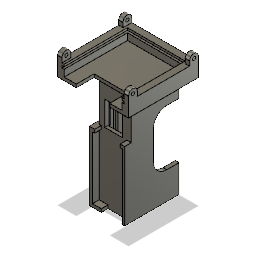
TinyTrack v7 (Autodesk Fusion 360 design; units mm, degrees)
Autodesk Fusion 360 part; units mm, degrees
sketch "Sketch1" plane through (0, 0, 0) normal (0, 1, 0) x (1, 0, 0)
  line L0 (0, 0) -> (26, 0)
  line L1 (26, 0) -> (26, 28.5)
  line L2 (26, 28.5) -> (0, 28.5)
  line L3 (0, 28.5) -> (0, 0)
  line L4 (29, -3) -> (29, 31.5)
  line L5 (29, 31.5) -> (-3, 31.5)
  line L6 (-3, 31.5) -> (-3, -3)
  line L7 (-3, -3) -> (29, -3)
  line L8 (27, -1) -> (27, 29.5)
  line L9 (27, 29.5) -> (-1, 29.5)
  line L10 (-1, 29.5) -> (-1, -1)
  line L11 (-1, -1) -> (27, -1)
  line L12 (-1, -1) -> (-1, -3)
  line L13 (27, -1) -> (27, -3)
  line L14 (0, 0) -> (0, -1)
  line L15 (26, 0) -> (26, -1)
  line L16 (0, -1) -> (0, -3)
  line L17 (26, -1) -> (26, -3)
  line L18 (5.5, -3) -> (20.5, -3)
  line L19 (20.5, -3) -> (20.5, 8)
  line L20 (20.5, 8) -> (5.5, 8)
  line L21 (5.5, 8) -> (5.5, -3)
  line L22 (7.5, 31.5) -> (18.5, 31.5)
  line L23 (18.5, 31.5) -> (18.5, 11.5)
  line L24 (18.5, 11.5) -> (7.5, 11.5)
  line L25 (7.5, 11.5) -> (7.5, 31.5)
  line L26 (20.25, 31.5) -> (20.25, 10)
  line L27 (20.25, 10) -> (5.75, 10)
  line L28 (5.75, 10) -> (5.75, 31.5)
  line L29 (26, 28.5) -> (26, 29.5)
  line L30 (0, 28.5) -> (0, 29.5)
  line L31 (7.5, 15.5) -> (8.75, 15.5)
  line L32 (8.75, 15.5) -> (8.75, 17.5)
  line L33 (8.75, 17.5) -> (7.5, 17.5)
  line L34 (7.5, 17.5) -> (7.5, 15.5)
  line L35 (18.5, 15.5) -> (17.25, 15.5)
  line L36 (17.25, 15.5) -> (17.25, 17.5)
  line L37 (17.25, 17.5) -> (18.5, 17.5)
  line L38 (18.5, 17.5) -> (18.5, 15.5)
  line L39 (7.5, 11.5) -> (8.75, 11.5)
  line L40 (8.75, 11.5) -> (8.75, 13.5)
  line L41 (8.75, 13.5) -> (7.5, 13.5)
  line L42 (7.5, 13.5) -> (7.5, 11.5)
  line L43 (18.5, 11.5) -> (17.25, 11.5)
  line L44 (17.25, 11.5) -> (17.25, 13.5)
  line L45 (17.25, 13.5) -> (18.5, 13.5)
  line L46 (18.5, 13.5) -> (18.5, 11.5)
  line L47 (26, 0) -> (29, 0)
  line L48 (0, 0) -> (-3, 0)
  dimension "d1" = 26
  dimension "d2" = 28.5
  dimension "d3" = 3
  dimension "d4" = 1
  dimension "d15" = 15
  dimension "d16" = 11
  dimension "d17" = 5.5
  dimension "d18" = 11
  dimension "d19" = 20
  dimension "d21" = 1.25
  dimension "d22" = 2
  dimension "d23" = 2
  dimension "d24" = 1.25
  dimension "d25" = 4
  dimension "d26" = 4
  dimension "d42" = 1.25
  dimension "d43" = 2
  dimension "d44" = 2
  dimension "d45" = 1.25
  dimension "d56" = 1.75
  dimension "d57" = 1.75
  dimension "d58" = 8.75
  measures "d17" distance of L3 L21
  measures "d25" distance of L24 L31
  measures "d26" distance of L24 L35
  measures "d56" distance of L23 L26
  measures "d57" distance of L25 L28
  measures "d58" distance of L4 L26
extrude "Extrude1" add sketch "Sketch1" along normal blind 1.5 contours L0 L1 L2 L3 L19 L20 L21 L26 L27 L28 | L2 L23 L24 L25 L26 L27 L28 L34 L38 L39 L42 L43 L46 | L2 L23 L24 L25 L31 L32 L33 L35 L36 L37 L40 L41 L44 L45 | L25 L31 L32 L33 L34 | L23 L35 L36 L37 L38 | L24 L25 L39 L40 L41 L42 | L23 L24 L43 L44 L45 L46
extrude "Extrude2" add sketch "Sketch1" along normal blind 4.5 contours L3 L9 L10 L30 L48 | L2 L9 L28 L30 | L2 L9 L25 L28 | L1 L8 L9 L29 L47 | L2 L9 L23 L25 | L2 L9 L26 L29 | L2 L9 L23 L26
extrude "Extrude3" add sketch "Sketch1" along normal blind 6.5 contours L5 L6 L9 L10 L28 L48 | L5 L9 L25 L28 | L4 L5 L8 L9 L26 L47 | L5 L9 L22 L23 L25 | L5 L9 L23 L26
extrude "Extrude4" add sketch "Sketch1" along normal blind 1 from surface at 5.5 contours L3 L9 L10 L30 L48 | L2 L9 L28 L30 | L2 L9 L25 L28 | L1 L8 L9 L29 L47 | L2 L9 L23 L25 | L2 L9 L26 L29 | L2 L9 L23 L26
extrude "Extrude5" add sketch "Sketch1" against normal blind 50 contours L2 L9 L25 L28 | L2 L23 L24 L25 L26 L27 L28 L34 L38 L39 L42 L43 L46 | L5 L9 L25 L28 | L2 L9 L23 L26 | L25 L31 L32 L33 L34 | L5 L9 L23 L26 | L23 L35 L36 L37 L38 | L24 L25 L39 L40 L41 L42 | L23 L24 L43 L44 L45 L46
sketch "Sketch2" plane through (20.25, 0, 0) normal (1, 0, 0) x (0, 0, -1)
  line L0 (31.5, 0) -> (10, 0)
  line L1 (10, 0) -> (10, -50)
  line L2 (10, -50) -> (31.5, -50)
  line L3 (31.5, -50) -> (31.5, 0)
  line L4 (31.5, -12.5) -> (26, -12.5)
  line L5 (20, -18.5) -> (20, -31.5)
  line L6 (26, -37.5) -> (31.5, -37.5)
  line L7 (31.5, -37.5) -> (31.5, -12.5)
  arc A0 (26, -12.5) -> (20, -18.5) centre (26, -18.5) ccw
  arc A1 (20, -31.5) -> (26, -37.5) centre (26, -31.5) ccw
  dimension "d29" = 25
  dimension "d30" = 11.5
  dimension "d31" = 12.5
  dimension "d32" = 6
  dimension "d33" = 6
  measures "d29" distance of L4 L6
  measures "d30" distance of L5 L7
  measures "d31" distance of L0 L4
  measures "d32" radius of A0
  measures "d33" radius of A1
extrude "Extrude6" cut sketch "Sketch2" against normal blind 15 contours L3 L4 L5 L6 L7 A0 A1
sketch "Sketch3" plane through (0, 0, -10) normal (0, 0, 1) x (1, 0, 0)
  line L0 (20.25, 0) -> (5.75, 0)
  line L1 (5.75, 0) -> (5.75, -50)
  line L2 (5.75, -50) -> (20.25, -50)
  line L3 (20.25, -50) -> (20.25, 0)
  line L4 (8.25, -8) -> (16.25, -8)
  line L5 (16.25, -8) -> (16.25, -19)
  line L6 (16.25, -19) -> (8.25, -19)
  line L7 (8.25, -19) -> (8.25, -8)
  line L8 (21, -50) -> (21, -22)
  line L9 (5.75, -22) -> (5.75, -50)
  line L10 (5.75, -48.5) -> (21, -48.5)
  line L11 (21, -48.5) -> (21, -20.5)
  line L12 (21, -20.5) -> (5.75, -20.5)
  line L13 (5.75, -20.5) -> (5.75, -48.5)
  line L14 (5.75, -19) -> (19.25, -19)
  line L15 (19.25, -19) -> (20.75, -19)
  line L16 (20.75, -19) -> (20.75, -50)
  line L17 (20.75, -50) -> (19.25, -50)
  line L18 (19.25, -50) -> (19.25, -19)
  line L19 (5.75, -19) -> (4.25, -19)
  line L20 (4.25, -19) -> (4.25, -50)
  line L21 (4.25, -50) -> (5.75, -50)
  line L22 (5.75, -50) -> (5.75, -19)
  line L23 (9.75, -48.5) -> (9.75, -50)
  line L24 (18.25, -19) -> (18.25, -20.5)
  line L25 (6.75, -19) -> (6.75, -20.5)
  dimension "d36" = 8
  dimension "d37" = 11
  dimension "d38" = 8
  dimension "d39" = 2.5
  dimension "d61" = 28
  dimension "d62" = 1.5
  dimension "d63" = 13.5
  dimension "d64" = 1.5
  dimension "d65" = 1.5
  dimension "d66" = 1.5
  dimension "d67" = 1
  dimension "d69" = 1
  measures "d38" distance of L0 L4
  measures "d39" distance of L1 L7
  measures "d62" distance of L2 L10
  measures "d64" distance of L12 L14
  measures "d67" distance of L18 L24
  measures "d69" distance of L22 L25
extrude "Extrude7" cut sketch "Sketch3" against normal blind 2 contours L4 L5 L6 L7 L14
extrude "Extrude8" add sketch "Sketch3" against normal blind 2 contours L1 L12 L14 L22 L25 | L1 L9 L13 L19 L20 L21 L22 | L12 L14 L18 L24 | L1 L2 L9 L10 L22 L23
extrude "Extrude9" add sketch "Sketch3" along normal blind 3 contours L3 L12 L15 L18 | L1 L12 L14 L22 L25 | L1 L9 L13 L19 L20 L21 L22 | L3 L10 L12 L18 | L12 L14 L18 L24 | L2 L3 L10 L17 L18 | L1 L2 L9 L10 L22 L23
sketch "Sketch4" plane through (-3, 0, 0) normal (-1, 0, 0) x (0, 0, 1)
  line L0 (-31.5, 0) -> (0, 0)
  line L1 (0, 0) -> (0, 6.5)
  line L2 (0, 6.5) -> (-31.5, 6.5)
  line L3 (-31.5, 6.5) -> (-31.5, 0)
  line L4 (-31.5, 6.5) -> (-27.5, 6.5)
  line L5 (-27.5, 6.5) -> (-27.5, 8.5)
  line L6 (-31.5, 8.5) -> (-31.5, 8.5)
  line L7 (-31.5, 7.5) -> (-31.5, 6.5)
  line L8 (0, 6.5) -> (-4, 6.5)
  line L9 (-4, 6.5) -> (-4, 8.5)
  line L10 (-4, 8.4862) -> (-4, 8.4862)
  line L11 (0, 8.5) -> (0, 6.5)
  circle A0 centre (-29.5, 8.5) radius 0.75
  arc A1 (-27.5, 8.5) -> (-31.5, 8.5) centre (-29.5, 8.5) ccw
  arc A2 (0, 8.5) -> (-4, 8.4862) centre (-2, 8.5) ccw
  circle A3 centre (-2, 8.5) radius 0.75
  line L12 (-31.5, 7.5) -> (-31.5, 8.5)
  arc A4 (0, 8.5) -> (-4, 8.5) centre (-2, 8.5) ccw
  dimension "d75" = 4
  dimension "d76" = 4
  dimension "d77" = 4
  dimension "d78" = 4
  dimension "d79" = 1.5
  dimension "d82" = 2
  dimension "d83" = 2
  dimension "d99" = 1.5
  dimension "d100" = 2
  dimension "d101" = 2
  dimension "d102" = 2
  dimension "d103" = 2
  measures "d79" diameter of A0
  measures "d82" radius of A1
  measures "d83" radius of A2
  measures "d99" diameter of A3
  measures "d100" distance of L2
  measures "d101" distance of L2
  measures "d102" distance of L2
  measures "d103" distance of L2
extrude "Extrude10" add sketch "Sketch4" against normal blind 2 contours L2 L4 L5 L7 A1 L12 | L2 L8 L9 L11 A2 A4
sketch "Sketch5" plane through (29, 0, 0) normal (1, 0, 0) x (0, 0, -1)
  line L0 (0, 0) -> (31.5, 0)
  line L1 (31.5, 0) -> (31.5, 6.5)
  line L2 (31.5, 6.5) -> (0, 6.5)
  line L3 (0, 6.5) -> (0, 0)
  line L4 (0, 6.5) -> (4, 6.5)
  line L5 (4, 6.5) -> (4, 8.5)
  line L6 (1.9875, 10.5) -> (1.9875, 10.5)
  line L7 (0, 8.5) -> (0, 6.5)
  line L8 (31.5, 6.5) -> (27.5, 6.5)
  line L9 (27.5, 6.5) -> (27.5, 8.5)
  line L10 (29.4713, 10.4998) -> (29.4713, 10.4998)
  line L11 (31.5, 8.5) -> (31.5, 6.5)
  circle A0 centre (29.5, 8.5) radius 0.75
  circle A1 centre (2, 8.5) radius 0.75
  arc A2 (1.9875, 10.5) -> (0, 8.5) centre (2, 8.5) ccw
  arc A3 (4, 8.5) -> (1.9875, 10.5) centre (2, 8.5) ccw
  arc A4 (29.4713, 10.4998) -> (27.5, 8.5) centre (29.5, 8.5) ccw
  arc A5 (31.5, 8.5) -> (29.4713, 10.4998) centre (29.5, 8.5) ccw
  dimension "d87" = 4
  dimension "d88" = 4
  dimension "d89" = 4
  dimension "d90" = 4
  dimension "d91" = 1.5
  dimension "d92" = 1.5
  dimension "d93" = 2
  dimension "d94" = 2
  dimension "d95" = 2
  dimension "d96" = 2
  dimension "d104" = 2
  dimension "d105" = 2
  dimension "d106" = 2
  dimension "d107" = 2
  measures "d91" diameter of A0
  measures "d92" diameter of A1
  measures "d93" radius of A2
  measures "d94" radius of A3
  measures "d95" radius of A4
  measures "d96" radius of A5
  measures "d104" distance of L2
  measures "d105" distance of L2
  measures "d106" distance of L4
  measures "d107" distance of L4
extrude "Extrude11" add sketch "Sketch5" against normal blind 2 contours L2 L4 L5 L7 A2 A3 | L2 L8 L9 L11 A4 A5
named bodies: "TinyTrack"
